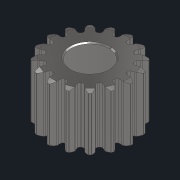
# Autodesk Inventor part: GEAHBB1_0-16-12-A-8_b
Saved by Autodesk Inventor 2022 (Build 260153000, 153)
## iProperties
Category: PARTsolutions
Company: MISUMI
Part Number: GEAHBB1_0-16-12-A-8_b
Material: 鋼、炭素鋼
Catalog Web Link: www.cadenas.de
Description: GEAHB1.0, GEAHBB1.0, GEAHBG1.0, GEAHS1.0, GEAB1.0, GEABB1.0, GEABG1.0, GEAS1.0, GEAKB1.0, GEAKBB1.0, GEAKBG1.0, GEAKS1.0_body-Spur Gears - Pressure Angle 20 Degree Module 1.0
Vendor: MISUMI
Document SubType Name: Modeling
Designer: partserver
Manufacturer: MISUMI
Mass: 13.5515 g
Surface Area: 17.3975 cm^2
Volume: 1.72631 cm^3
Density: 7.85 g/cm^3
Appearance: 半つや出し
PSOL_IDENT_0: {$CADENAS_DATA\23d-libs\misumi\metric\54_spur_gears\geab10\geab10.prj},528 {VTYP=3D},{NB=GEAHBB1.0-1
PSOL_IDENT_1: 6-12-A-8_b},{LINA=GEAHBB1.0-16-12-A-8},{NN=GEAHB1.0, GEAHBB1.0, GEAHBG1.0, GEAHS1.0, GEAB1.0, GEABB1
PSOL_IDENT_2: .0, GEABG1.0, GEAS1.0, GEAKB1.0, GEAKBB1.0, GEAKBG1.0, GEAKS1.0_body},{DATE=07.06.2021 01:25:53},{GE
PSOL_IDENT_3: OMDATE=08.04.2021 05:23:06},{VERSION=},{LINEID=20},{WBVAR=SHS,MAT,ST,NT,B,TSSE,TS,PS,ALT1,ALT2,TPC,A
PSOL_IDENT_4: LT11,ALT10,BS,ALT4,Z,J,ALT5,Q,R,S,T,ALT9,SRG,ALT6,LFC,LTC,MALT6,ALT7,KFC,KTC,K,ALT3,DIRALT3,QFC,QTC,
PSOL_IDENT_5: MALT3,ALT8,DIRALT8,ZFC,ZTC,U},{WBNUMERIC=NT,B,BS,Z,J,Q,R,S,T,SRG,LFC,LTC,KFC,KTC,K,QFC,QTC,ZFC,ZTC,U
PSOL_IDENT_6: }  {NB=GEAHBB1.0-16-12-A-8_b},{LINA=GEAHBB1.0-16-12-A-8},{KT=DUMMY},{PN=GEAHBB1.0-16-12-A-8},{SHS=RH
PSOL_IDENT_7: },{TYPE=GEAHBB},{MAT=S45C},{MATALG= 'S45C','S45C Equivalent','SUS304','SUS304' },{ST=BO},{STALG= '','
PSOL_IDENT_8: -','BO','Black Oxide','ENP','Electroless Nickel Plating'},{AC=-},{MOD=1.0},{NT=16},{NTALG=12,13,14,1
PSOL_IDENT_9: 5,16,17,18,19,20,21,22,23,24,25,26,27,28,29,30,32,33,34,35,36,38,39,40,42,44,45,46,48,49,50,51,52,54
PSOL_IDENT_10: ,55,56,57,58,60,62,63,64,65,66,68,69,70,72,75,76,77,78,80,81,84,85,88,90,91,92,95,96,98,99,100,110,1
PSOL_IDENT_11: 20},{B=12},{BALG=6,8,10,12},{TSSE=TSSE},{TSSEALG= '','Not Specified','TSSE','Specified'},{TS=A},{TSA
PSOL_IDENT_12: LG='K','K','A','A'},{TSPN=-A},{PS=8},{PSALG='6','6','6.35','6.35','7','7','8','8','9','9','10','10','
PSOL_IDENT_13: 11','11','12','12'},{P=8.00},{DD=16},{D=18},{G=13.5},{H=0},{L=0},{LL1=0},{LL2=0},{M=-},{ML=0.000},{A
PSOL_IDENT_14: LT1=},{ALT1ALG= '','N/A' },{ALT1PN=},{KC=0},{ALT2=},{ALT2ALG= '','N/A' },{TPC=N/A},{TPCALG= 'N/A' },
PSOL_IDENT_15: {ALT2PN=},{ALT11=},{ALT11ALG= '','N/A' },{ALT11PN=},{DEG=0},{ALT10=},{ALT10ALG= '','Not applicable'
PSOL_IDENT_16: },{BS=0.0},{BSALG=0},{BSMIN=3},{BSMAX=0},{ALT10PN=},{LL13D=0},{LL23D=0},{LBS=12},{ALT4=},{ALT4ALG=''
PSOL_IDENT_17: ,'Not applicable'},{ALT41=0},{ALT42=0},{ALT4PN=},{Z=0},{ZALG=0},{ZPN=},{ZMINL=10},{ZMAXL=9},{ZMINR=1
PSOL_IDENT_18: 0},{ZMAXR=9},{J=0.0},{JALG=0},{JPN=},{JMIN=2.0},{JMAX=0.0},{ALT5=},{ALT5ALG= '','Not applicable' },{
PSOL_IDENT_19: ALT5PN=},{Q=0},{QALG=0},{QPN=},{QMIN=10},{QMAX=9},{R=0},{RALG=0},{RPN=},{RMIN=10},{RMAX=9.0},{S=0},{
PSOL_IDENT_20: SALG=0},{SPN=},{SMIN=3},{SMAX=6},{T=0},{TALG=0},{TPN=},{TMIN=3},{TMAX=0},{ALT9=},{ALT9ALG= '','Not a
PSOL_IDENT_21: pplicable' },{SRG=0.0},{SRGALG=0},{SRGMIN=3.500},{SRGMINALG=3.500},{SRGMAX=0.000},{SRGMAXALG=0.000},
PSOL_IDENT_22: {DD2=0.0},{MM=0.00},{NN=0.00},{DD2ALG=0.000},{MMALG=0.000},{NNALG=0.000},{ALT9PN=},{ALT6=},{ALT6ALG=
PSOL_IDENT_23: '','Not applicable' },{ALT6PN=},{LFC=0},{LFCALG=0},{LTC=0},{LTCALG=0},{LPCDMIN=16},{LPCDMAX=6},{MAL
PSOL_IDENT_24: T6=N/A},{MALT6ALG= 'N/A' },{C=0.0},{ALT7=},{ALT7ALG= '','Not applicable' },{ALT7PN=},{KFC=0},{KFCALG=
PSOL_IDENT_25: [0]},{KTC=0},{KTCALG=[0]},{KPCDMIN1=15},{KPCDMAX1=-7},{KPCDMIN2=7},{KPCDMAX2=6},{KPCD=0},{K=0.0},{KA
PSOL_IDENT_26: LG=[0]},{KALT7L=12},{SCREW=0},{SCREWL=0},{ALT3=},{ALT3ALG= '','Not applicable' },{DIRALT3=},{DIRALT3
PSOL_IDENT_27: ALG= '','N/A' },{ALT3PN=},{QFC=0},{QFCALG=[0]},{QTC=0},{QTCALG=[0]},{QPCDMIN1=15},{QPCDMAX1=-7},{QPC
PSOL_IDENT_28: DMIN2=7},{QPCDMAX2=6},{CIFMALT3=3},{QPCD=0},{MALT3=N/A},{MALT3ALG= 'N/A' },{MALT3L=0},{MS1=3},{PITCH=
PSOL_IDENT_29: 0},{BB=3},{TT=0},{ALT8=},{ALT8ALG= '','Not applicable' },{DIRALT8=},{DIRALT8ALG= '','N/A' },{ALT8PN=
PSOL_IDENT_30: },{ZFC=0},{ZFCALG=[0]},{ZFCMIN=18},{ZFCMAX=3},{ZTC=0},{ZTCALG=[0]},{ZPCDMIN1=18},{ZPCDMIN2=11},{ZPCD
PSOL_IDENT_31: MAX1=-10},{ZPCDMAX2=3},{ZPCD=0},{U=0},{UALG=[0]},{UMAX=0},{UMAX1=0},{UMAX2=5},{UMIN=3},{U1=0.0},{U2=
PSOL_IDENT_32: 0.0},{F=0.0},{PLANE=4},{BL1=12},{BL2=11.5},{PCD=0},{SHN=0},{SHDEG1=0},{SHDEG2=0},{PZQRDD2=8},{ALT3LB
PSOL_IDENT_33: S=11.5},{D1=5.625},{D2=11.25},{D3=20},{D4=0.1},{D5=2.666667},{D6=2.461538},{D7=0.85},{D8=0.5},{D9=0.
PSOL_IDENT_34: 809481},{S1=15},{S2=1},{KR=22.5}
NB: GEAHBB1.0-16-12-A-8_b
NN: 0
NT: 16
NBSYN: $PN._b
LINA: GEAHBB1.0-16-12-A-8
CATALOG: Misumi
PN: GEAHBB1.0-16-12-A-8
SHS: Round Hole
MAT: S45C Equivalent
ST: Black Oxide
AC: -
MOD: 1
B: 12
TSSE: Specified
TS: A
PS: 8
DD: 16
D: 18
G: 13.5
H: 0
L: 0
LL1: 0
LL2: 0
M: -
ALT1: N/A
ALT2: N/A
TPC: N/A
ALT11: N/A
ALT10: Not applicable
BS: 0
ALT4: Not applicable
Z: 0
J: 0
ALT5: Not applicable
Q: 0
R: 0
S: 0
T: 0
ALT9: Not applicable
SRG: 0
DD2: 0
MM: 0
ALT6: Not applicable
LFC: 0
LTC: 0
MALT6: N/A
C: 0
ALT7: Not applicable
KFC: 0
KTC: 0
K: 0
ALT3: Not applicable
DIRALT3: N/A
QFC: 0
QTC: 0
MALT3: N/A
ALT8: Not applicable
DIRALT8: N/A
ZFC: 0
ZTC: 0
U: 0
U1: 0
U2: 0
F: 0
SUPPLIER: MISUMI
ARTICLENO: GEAHBB1.0-16-12-A-8_b
BOMINFO: GEAHBB1.0-16-12-A-8
CREATOR: CADENAS GmbH
Title: GEAHBB1.0-16-12-A-8
Author: Cadenas PARTsolutions
Comments: Spur Gears - Pressure Angle 20 Degree Module 1.0
Autodesk Inventor part; units mm, degrees
sketch "Sketch_12" plane through (0, 0, 0) normal (1, 0, 0) x (0, 1, 0)
  line L0 (0, 0) -> (0, 12)
  line L1 (0, 12) -> (8, 12)
  line L2 (8, 12) -> (14, 10.3923)
  line L3 (14, 10.3923) -> (14, 1.6077)
  line L4 (14, 1.6077) -> (8, 0)
  line L5 (8, 0) -> (0, 0)
  line L6 (0, 0) -> (0, 12)
  constraints: 14 end point
revolve "Revolution1" add sketch "Sketch_12" angle 360 about axis through (0, 0, 0) along (0, 0, -1)
sketch "Sketch_3" plane through (0, 0, 0) normal (0, 0, 1) x (1, 0, 0)
  circle A0 centre (0, 0) radius 36
  arc A1 (-8.9975, 0.2118) -> (-8.9975, -0.2118) centre (0, 0) ccw
  arc A2 (-8.9975, -0.2118) -> (-8.9598, -0.2877) centre (-8.8975, -0.2094) ccw
  arc A3 (-8.9598, -0.2877) -> (-7.9615, -0.7841) centre (-7.2994, 1.799) ccw
  arc A4 (-7.9615, -0.7841) -> (-7.6733, -0.8048) centre (-7.7605, 0) ccw
  arc A5 (-7.06, -0.8151) -> (-7.6733, -0.8048) centre (-7.4079, -3.252) ccw
  arc A6 (-6.6389, -1.2198) -> (-7.06, -0.8151) centre (-7.1306, -1.3101) ccw
  arc A7 (-6.6389, -1.2198) -> (-6.6003, -1.4137) centre (0, 0) ccw
  arc A8 (-6.8345, -1.9486) -> (-6.6003, -1.4137) centre (-7.0892, -1.5184) ccw
  arc A9 (-7.3971, -2.1929) -> (-6.8345, -1.9486) centre (-8.0885, 0.1695) ccw
  arc A10 (-7.3971, -2.1929) -> (-7.6555, -2.3223) centre (-7.1698, -2.9698) ccw
  arc A11 (-7.6555, -2.3223) -> (-8.3879, -3.163) centre (-6.0553, -4.4555) ccw
  arc A12 (-8.3879, -3.163) -> (-8.3936, -3.2476) centre (-8.3004, -3.2115) ccw
  arc A13 (-8.3936, -3.2476) -> (-8.2316, -3.6388) centre (0, 0) ccw
  arc A14 (-8.2316, -3.6388) -> (-8.1677, -3.6945) centre (-8.1401, -3.5984) ccw
  arc A15 (-8.1677, -3.6945) -> (-7.0554, -3.7712) centre (-7.4323, -1.1313) ccw
  arc A16 (-7.0554, -3.7712) -> (-6.7812, -3.6799) centre (-7.1698, -2.9698) ccw
  arc A17 (-6.2106, -3.4548) -> (-6.7812, -3.6799) centre (-5.5995, -5.8393) ccw
  arc A18 (-5.6667, -3.6675) -> (-6.2106, -3.4548) centre (-6.0865, -3.9392) ccw
  arc A19 (-5.6667, -3.6675) -> (-5.5569, -3.8319) centre (0, 0) ccw
  arc A20 (-5.5685, -4.4158) -> (-5.5569, -3.8319) centre (-5.9685, -4.1157) ccw
  arc A21 (-5.9949, -4.8568) -> (-5.5685, -4.4158) centre (-7.5377, -2.9387) ccw
  arc A22 (-5.9949, -4.8568) -> (-6.1841, -5.0751) centre (-5.4875, -5.4875) ccw
  arc A23 (-6.1841, -5.0751) -> (-6.5389, -6.1321) centre (-3.8894, -6.4336) ccw
  arc A24 (-6.5389, -6.1321) -> (-6.5119, -6.2125) centre (-6.4396, -6.1434) ccw
  arc A25 (-6.5119, -6.2125) -> (-6.2125, -6.5119) centre (0, 0) ccw
  arc A26 (-6.2125, -6.5119) -> (-6.1321, -6.5389) centre (-6.1434, -6.4396) ccw
  arc A27 (-6.1321, -6.5389) -> (-5.0751, -6.1841) centre (-6.4336, -3.8894) ccw
  arc A28 (-5.0751, -6.1841) -> (-4.8568, -5.9949) centre (-5.4875, -5.4875) ccw
  arc A29 (-4.4158, -5.5685) -> (-4.8568, -5.9949) centre (-2.9387, -7.5377) ccw
  arc A30 (-3.8319, -5.5569) -> (-4.4158, -5.5685) centre (-4.1157, -5.9685) ccw
  arc A31 (-3.8319, -5.5569) -> (-3.6675, -5.6667) centre (0, 0) ccw
  arc A32 (-3.4548, -6.2106) -> (-3.6675, -5.6667) centre (-3.9392, -6.0865) ccw
  arc A33 (-3.6799, -6.7812) -> (-3.4548, -6.2106) centre (-5.8393, -5.5995) ccw
  arc A34 (-3.6799, -6.7812) -> (-3.7712, -7.0554) centre (-2.9698, -7.1698) ccw
  arc A35 (-3.7712, -7.0554) -> (-3.6945, -8.1677) centre (-1.1313, -7.4323) ccw
  arc A36 (-3.6945, -8.1677) -> (-3.6388, -8.2316) centre (-3.5984, -8.1401) ccw
  arc A37 (-3.6388, -8.2316) -> (-3.2476, -8.3936) centre (0, 0) ccw
  arc A38 (-3.2476, -8.3936) -> (-3.163, -8.3879) centre (-3.2115, -8.3004) ccw
  arc A39 (-3.163, -8.3879) -> (-2.3223, -7.6555) centre (-4.4555, -6.0553) ccw
  arc A40 (-2.3223, -7.6555) -> (-2.1929, -7.3971) centre (-2.9698, -7.1698) ccw
  arc A41 (-1.9486, -6.8345) -> (-2.1929, -7.3971) centre (0.1695, -8.0885) ccw
  arc A42 (-1.4137, -6.6003) -> (-1.9486, -6.8345) centre (-1.5184, -7.0892) ccw
  arc A43 (-1.4137, -6.6003) -> (-1.2198, -6.6389) centre (0, 0) ccw
  arc A44 (-0.8151, -7.06) -> (-1.2198, -6.6389) centre (-1.3101, -7.1306) ccw
  arc A45 (-0.8048, -7.6733) -> (-0.8151, -7.06) centre (-3.252, -7.4079) ccw
  arc A46 (-0.8048, -7.6733) -> (-0.7841, -7.9615) centre (0, -7.7605) ccw
  arc A47 (-0.7841, -7.9615) -> (-0.2877, -8.9598) centre (1.799, -7.2994) ccw
  arc A48 (-0.2877, -8.9598) -> (-0.2118, -8.9975) centre (-0.2094, -8.8975) ccw
  arc A49 (-0.2118, -8.9975) -> (0.2118, -8.9975) centre (0, 0) ccw
  arc A50 (0.2118, -8.9975) -> (0.2877, -8.9598) centre (0.2094, -8.8975) ccw
  arc A51 (0.2877, -8.9598) -> (0.7841, -7.9615) centre (-1.799, -7.2994) ccw
  arc A52 (0.7841, -7.9615) -> (0.8048, -7.6733) centre (0, -7.7605) ccw
  arc A53 (0.8151, -7.06) -> (0.8048, -7.6733) centre (3.252, -7.4079) ccw
  arc A54 (1.2198, -6.6389) -> (0.8151, -7.06) centre (1.3101, -7.1306) ccw
  arc A55 (1.2198, -6.6389) -> (1.4137, -6.6003) centre (0, 0) ccw
  arc A56 (1.9486, -6.8345) -> (1.4137, -6.6003) centre (1.5184, -7.0892) ccw
  arc A57 (2.1929, -7.3971) -> (1.9486, -6.8345) centre (-0.1695, -8.0885) ccw
  arc A58 (2.1929, -7.3971) -> (2.3223, -7.6555) centre (2.9698, -7.1698) ccw
  arc A59 (2.3223, -7.6555) -> (3.163, -8.3879) centre (4.4555, -6.0553) ccw
  arc A60 (3.163, -8.3879) -> (3.2476, -8.3936) centre (3.2115, -8.3004) ccw
  arc A61 (3.2476, -8.3936) -> (3.6388, -8.2316) centre (0, 0) ccw
  arc A62 (3.6388, -8.2316) -> (3.6945, -8.1677) centre (3.5984, -8.1401) ccw
  arc A63 (3.6945, -8.1677) -> (3.7712, -7.0554) centre (1.1313, -7.4323) ccw
  arc A64 (3.7712, -7.0554) -> (3.6799, -6.7812) centre (2.9698, -7.1698) ccw
  arc A65 (3.4548, -6.2106) -> (3.6799, -6.7812) centre (5.8393, -5.5995) ccw
  arc A66 (3.6675, -5.6667) -> (3.4548, -6.2106) centre (3.9392, -6.0865) ccw
  arc A67 (3.6675, -5.6667) -> (3.8319, -5.5569) centre (0, 0) ccw
  arc A68 (4.4158, -5.5685) -> (3.8319, -5.5569) centre (4.1157, -5.9685) ccw
  arc A69 (4.8568, -5.9949) -> (4.4158, -5.5685) centre (2.9387, -7.5377) ccw
  arc A70 (4.8568, -5.9949) -> (5.0751, -6.1841) centre (5.4875, -5.4875) ccw
  arc A71 (5.0751, -6.1841) -> (6.1321, -6.5389) centre (6.4336, -3.8894) ccw
  arc A72 (6.1321, -6.5389) -> (6.2125, -6.5119) centre (6.1434, -6.4396) ccw
  arc A73 (6.2125, -6.5119) -> (6.5119, -6.2125) centre (0, 0) ccw
  arc A74 (6.5119, -6.2125) -> (6.5389, -6.1321) centre (6.4396, -6.1434) ccw
  arc A75 (6.5389, -6.1321) -> (6.1841, -5.0751) centre (3.8894, -6.4336) ccw
  arc A76 (6.1841, -5.0751) -> (5.9949, -4.8568) centre (5.4875, -5.4875) ccw
  arc A77 (5.5685, -4.4158) -> (5.9949, -4.8568) centre (7.5377, -2.9387) ccw
  arc A78 (5.5569, -3.8319) -> (5.5685, -4.4158) centre (5.9685, -4.1157) ccw
  arc A79 (5.5569, -3.8319) -> (5.6667, -3.6675) centre (0, 0) ccw
  arc A80 (6.2106, -3.4548) -> (5.6667, -3.6675) centre (6.0865, -3.9392) ccw
  arc A81 (6.7812, -3.6799) -> (6.2106, -3.4548) centre (5.5995, -5.8393) ccw
  arc A82 (6.7812, -3.6799) -> (7.0554, -3.7712) centre (7.1698, -2.9698) ccw
  arc A83 (7.0554, -3.7712) -> (8.1677, -3.6945) centre (7.4323, -1.1313) ccw
  arc A84 (8.1677, -3.6945) -> (8.2316, -3.6388) centre (8.1401, -3.5984) ccw
  arc A85 (8.2316, -3.6388) -> (8.3936, -3.2476) centre (0, 0) ccw
  arc A86 (8.3936, -3.2476) -> (8.3879, -3.163) centre (8.3004, -3.2115) ccw
  arc A87 (8.3879, -3.163) -> (7.6555, -2.3223) centre (6.0553, -4.4555) ccw
  arc A88 (7.6555, -2.3223) -> (7.3971, -2.1929) centre (7.1698, -2.9698) ccw
  arc A89 (6.8345, -1.9486) -> (7.3971, -2.1929) centre (8.0885, 0.1695) ccw
  arc A90 (6.6003, -1.4137) -> (6.8345, -1.9486) centre (7.0892, -1.5184) ccw
  arc A91 (6.6003, -1.4137) -> (6.6389, -1.2198) centre (0, 0) ccw
  arc A92 (7.06, -0.8151) -> (6.6389, -1.2198) centre (7.1306, -1.3101) ccw
  arc A93 (7.6733, -0.8048) -> (7.06, -0.8151) centre (7.4079, -3.252) ccw
  arc A94 (7.6733, -0.8048) -> (7.9615, -0.7841) centre (7.7605, 0) ccw
  arc A95 (7.9615, -0.7841) -> (8.9598, -0.2877) centre (7.2994, 1.799) ccw
  arc A96 (8.9598, -0.2877) -> (8.9975, -0.2118) centre (8.8975, -0.2094) ccw
  arc A97 (8.9975, -0.2118) -> (8.9975, 0.2118) centre (0, 0) ccw
  arc A98 (8.9975, 0.2118) -> (8.9598, 0.2877) centre (8.8975, 0.2094) ccw
  arc A99 (8.9598, 0.2877) -> (7.9615, 0.7841) centre (7.2994, -1.799) ccw
  arc A100 (7.9615, 0.7841) -> (7.6733, 0.8048) centre (7.7605, 0) ccw
  arc A101 (7.06, 0.8151) -> (7.6733, 0.8048) centre (7.4079, 3.252) ccw
  arc A102 (6.6389, 1.2198) -> (7.06, 0.8151) centre (7.1306, 1.3101) ccw
  arc A103 (6.6389, 1.2198) -> (6.6003, 1.4137) centre (0, 0) ccw
  arc A104 (6.8345, 1.9486) -> (6.6003, 1.4137) centre (7.0892, 1.5184) ccw
  arc A105 (7.3971, 2.1929) -> (6.8345, 1.9486) centre (8.0885, -0.1695) ccw
  arc A106 (7.3971, 2.1929) -> (7.6555, 2.3223) centre (7.1698, 2.9698) ccw
  arc A107 (7.6555, 2.3223) -> (8.3879, 3.163) centre (6.0553, 4.4555) ccw
  arc A108 (8.3879, 3.163) -> (8.3936, 3.2476) centre (8.3004, 3.2115) ccw
  arc A109 (8.3936, 3.2476) -> (8.2316, 3.6388) centre (0, 0) ccw
  arc A110 (8.2316, 3.6388) -> (8.1677, 3.6945) centre (8.1401, 3.5984) ccw
  arc A111 (8.1677, 3.6945) -> (7.0554, 3.7712) centre (7.4323, 1.1313) ccw
  arc A112 (7.0554, 3.7712) -> (6.7812, 3.6799) centre (7.1698, 2.9698) ccw
  arc A113 (6.2106, 3.4548) -> (6.7812, 3.6799) centre (5.5995, 5.8393) ccw
  arc A114 (5.6667, 3.6675) -> (6.2106, 3.4548) centre (6.0865, 3.9392) ccw
  arc A115 (5.6667, 3.6675) -> (5.5569, 3.8319) centre (0, 0) ccw
  arc A116 (5.5685, 4.4158) -> (5.5569, 3.8319) centre (5.9685, 4.1157) ccw
  arc A117 (5.9949, 4.8568) -> (5.5685, 4.4158) centre (7.5377, 2.9387) ccw
  arc A118 (5.9949, 4.8568) -> (6.1841, 5.0751) centre (5.4875, 5.4875) ccw
  arc A119 (6.1841, 5.0751) -> (6.5389, 6.1321) centre (3.8894, 6.4336) ccw
  arc A120 (6.5389, 6.1321) -> (6.5119, 6.2125) centre (6.4396, 6.1434) ccw
  arc A121 (6.5119, 6.2125) -> (6.2125, 6.5119) centre (0, 0) ccw
  arc A122 (6.2125, 6.5119) -> (6.1321, 6.5389) centre (6.1434, 6.4396) ccw
  arc A123 (6.1321, 6.5389) -> (5.0751, 6.1841) centre (6.4336, 3.8894) ccw
  arc A124 (5.0751, 6.1841) -> (4.8568, 5.9949) centre (5.4875, 5.4875) ccw
  arc A125 (4.4158, 5.5685) -> (4.8568, 5.9949) centre (2.9387, 7.5377) ccw
  arc A126 (3.8319, 5.5569) -> (4.4158, 5.5685) centre (4.1157, 5.9685) ccw
  arc A127 (3.8319, 5.5569) -> (3.6675, 5.6667) centre (0, 0) ccw
  arc A128 (3.4548, 6.2106) -> (3.6675, 5.6667) centre (3.9392, 6.0865) ccw
  arc A129 (3.6799, 6.7812) -> (3.4548, 6.2106) centre (5.8393, 5.5995) ccw
  arc A130 (3.6799, 6.7812) -> (3.7712, 7.0554) centre (2.9698, 7.1698) ccw
  arc A131 (3.7712, 7.0554) -> (3.6945, 8.1677) centre (1.1313, 7.4323) ccw
  arc A132 (3.6945, 8.1677) -> (3.6388, 8.2316) centre (3.5984, 8.1401) ccw
  arc A133 (3.6388, 8.2316) -> (3.2476, 8.3936) centre (0, 0) ccw
  arc A134 (3.2476, 8.3936) -> (3.163, 8.3879) centre (3.2115, 8.3004) ccw
  arc A135 (3.163, 8.3879) -> (2.3223, 7.6555) centre (4.4555, 6.0553) ccw
  arc A136 (2.3223, 7.6555) -> (2.1929, 7.3971) centre (2.9698, 7.1698) ccw
  arc A137 (1.9486, 6.8345) -> (2.1929, 7.3971) centre (-0.1695, 8.0885) ccw
  arc A138 (1.4137, 6.6003) -> (1.9486, 6.8345) centre (1.5184, 7.0892) ccw
  arc A139 (1.4137, 6.6003) -> (1.2198, 6.6389) centre (0, 0) ccw
  arc A140 (0.8151, 7.06) -> (1.2198, 6.6389) centre (1.3101, 7.1306) ccw
  arc A141 (0.8048, 7.6733) -> (0.8151, 7.06) centre (3.252, 7.4079) ccw
  arc A142 (0.8048, 7.6733) -> (0.7841, 7.9615) centre (0, 7.7605) ccw
  arc A143 (0.7841, 7.9615) -> (0.2877, 8.9598) centre (-1.799, 7.2994) ccw
  arc A144 (0.2877, 8.9598) -> (0.2118, 8.9975) centre (0.2094, 8.8975) ccw
  arc A145 (0.2118, 8.9975) -> (-0.2118, 8.9975) centre (0, 0) ccw
  arc A146 (-0.2118, 8.9975) -> (-0.2877, 8.9598) centre (-0.2094, 8.8975) ccw
  arc A147 (-0.2877, 8.9598) -> (-0.7841, 7.9615) centre (1.799, 7.2994) ccw
  arc A148 (-0.7841, 7.9615) -> (-0.8048, 7.6733) centre (0, 7.7605) ccw
  arc A149 (-0.8151, 7.06) -> (-0.8048, 7.6733) centre (-3.252, 7.4079) ccw
  arc A150 (-1.2198, 6.6389) -> (-0.8151, 7.06) centre (-1.3101, 7.1306) ccw
  arc A151 (-1.2198, 6.6389) -> (-1.4137, 6.6003) centre (0, 0) ccw
  arc A152 (-1.9486, 6.8345) -> (-1.4137, 6.6003) centre (-1.5184, 7.0892) ccw
  arc A153 (-2.1929, 7.3971) -> (-1.9486, 6.8345) centre (0.1695, 8.0885) ccw
  arc A154 (-2.1929, 7.3971) -> (-2.3223, 7.6555) centre (-2.9698, 7.1698) ccw
  arc A155 (-2.3223, 7.6555) -> (-3.163, 8.3879) centre (-4.4555, 6.0553) ccw
  arc A156 (-3.163, 8.3879) -> (-3.2476, 8.3936) centre (-3.2115, 8.3004) ccw
  arc A157 (-3.2476, 8.3936) -> (-3.6388, 8.2316) centre (0, 0) ccw
  arc A158 (-3.6388, 8.2316) -> (-3.6945, 8.1677) centre (-3.5984, 8.1401) ccw
  arc A159 (-3.6945, 8.1677) -> (-3.7712, 7.0554) centre (-1.1313, 7.4323) ccw
  arc A160 (-3.7712, 7.0554) -> (-3.6799, 6.7812) centre (-2.9698, 7.1698) ccw
  arc A161 (-3.4548, 6.2106) -> (-3.6799, 6.7812) centre (-5.8393, 5.5995) ccw
  arc A162 (-3.6675, 5.6667) -> (-3.4548, 6.2106) centre (-3.9392, 6.0865) ccw
  arc A163 (-3.6675, 5.6667) -> (-3.8319, 5.5569) centre (0, 0) ccw
  arc A164 (-4.4158, 5.5685) -> (-3.8319, 5.5569) centre (-4.1157, 5.9685) ccw
  arc A165 (-4.8568, 5.9949) -> (-4.4158, 5.5685) centre (-2.9387, 7.5377) ccw
  arc A166 (-4.8568, 5.9949) -> (-5.0751, 6.1841) centre (-5.4875, 5.4875) ccw
  arc A167 (-5.0751, 6.1841) -> (-6.1321, 6.5389) centre (-6.4336, 3.8894) ccw
  arc A168 (-6.1321, 6.5389) -> (-6.2125, 6.5119) centre (-6.1434, 6.4396) ccw
  arc A169 (-6.2125, 6.5119) -> (-6.5119, 6.2125) centre (0, 0) ccw
  arc A170 (-6.5119, 6.2125) -> (-6.5389, 6.1321) centre (-6.4396, 6.1434) ccw
  arc A171 (-6.5389, 6.1321) -> (-6.1841, 5.0751) centre (-3.8894, 6.4336) ccw
  arc A172 (-6.1841, 5.0751) -> (-5.9949, 4.8568) centre (-5.4875, 5.4875) ccw
  arc A173 (-5.5685, 4.4158) -> (-5.9949, 4.8568) centre (-7.5377, 2.9387) ccw
  arc A174 (-5.5569, 3.8319) -> (-5.5685, 4.4158) centre (-5.9685, 4.1157) ccw
  arc A175 (-5.5569, 3.8319) -> (-5.6667, 3.6675) centre (0, 0) ccw
  arc A176 (-6.2106, 3.4548) -> (-5.6667, 3.6675) centre (-6.0865, 3.9392) ccw
  arc A177 (-6.7812, 3.6799) -> (-6.2106, 3.4548) centre (-5.5995, 5.8393) ccw
  arc A178 (-6.7812, 3.6799) -> (-7.0554, 3.7712) centre (-7.1698, 2.9698) ccw
  arc A179 (-7.0554, 3.7712) -> (-8.1677, 3.6945) centre (-7.4323, 1.1313) ccw
  arc A180 (-8.1677, 3.6945) -> (-8.2316, 3.6388) centre (-8.1401, 3.5984) ccw
  arc A181 (-8.2316, 3.6388) -> (-8.3936, 3.2476) centre (0, 0) ccw
  arc A182 (-8.3936, 3.2476) -> (-8.3879, 3.163) centre (-8.3004, 3.2115) ccw
  arc A183 (-8.3879, 3.163) -> (-7.6555, 2.3223) centre (-6.0553, 4.4555) ccw
  arc A184 (-7.6555, 2.3223) -> (-7.3971, 2.1929) centre (-7.1698, 2.9698) ccw
  arc A185 (-6.8345, 1.9486) -> (-7.3971, 2.1929) centre (-8.0885, -0.1695) ccw
  arc A186 (-6.6003, 1.4137) -> (-6.8345, 1.9486) centre (-7.0892, 1.5184) ccw
  arc A187 (-6.6003, 1.4137) -> (-6.6389, 1.2198) centre (0, 0) ccw
  arc A188 (-7.06, 0.8151) -> (-6.6389, 1.2198) centre (-7.1306, 1.3101) ccw
  arc A189 (-7.6733, 0.8048) -> (-7.06, 0.8151) centre (-7.4079, 3.252) ccw
  arc A190 (-7.6733, 0.8048) -> (-7.9615, 0.7841) centre (-7.7605, 0) ccw
  arc A191 (-7.9615, 0.7841) -> (-8.9598, 0.2877) centre (-7.2994, -1.799) ccw
  arc A192 (-8.9598, 0.2877) -> (-8.9975, 0.2118) centre (-8.8975, 0.2094) ccw
  constraints: 384 point on circle, 193 centre point
extrude "Extrusion1" cut sketch "Sketch_3" along normal blind 13
sketch "Sketch3" plane through (0, 0, 0) normal (0, 0, -1) x (-1, 0, 0)
  point P0 (0, 0)
hole "Hole1" at (0, 0, 0) direction (0, 0, 1) diameter 8 depth 12
sketch "_____7" plane through (0, 0, 0) normal (1, 0, 0) x (0, 0, -1)
  line L0 (500, 0) -> (-500, 0)
  line L1 (-0.3, 4) -> (0, 4)
  line L2 (0, 4) -> (0, 4.3)
  line L3 (0, 4.3) -> (-0.3, 4)
  constraints: 8 end point
revolve "Revolution2" cut sketch "_____7" angle 360 about axis through (0, 0, -500) along (0, 0, -1)
sketch "_____17" plane through (0, 0, 0) normal (1, 0, 0) x (0, 0, -1)
  line L0 (500, 0) -> (-500, 0)
  line L1 (-12, 4.3) -> (-12, 4)
  line L2 (-12, 4) -> (-11.7, 4)
  line L3 (-11.7, 4) -> (-12, 4.3)
  constraints: 8 end point
revolve "Revolution3" cut sketch "_____17" angle 360 about axis through (0, 0, -500) along (0, 0, -1)
ref_plane "b_XY" through (0, 0, 0) normal (0, 0, 1) x (1, 0, 0)
ref_plane "b_YZ" through (0, 0, 0) normal (1, 0, 0) x (0, 1, 0)
ref_plane "b_ZX" through (0, 0, 0) normal (0, 1, 0) x (0, 0, 1)
ref_plane "turn_around_XY" through (0, 0, 0) normal (-1, 0, 0) x (0, 0, -1)
ref_plane "turn_around_YZ" through (0, 0, 0) normal (0, 0, -1) x (0, -1, 0)
ref_plane "turn_around_ZX" through (0, 0, 0) normal (0, -1, 0) x (-1, 0, 0)
sketch "スケッチ6" plane through (0, 0, 0) normal (0, 0, -1) x (-1, 0, 0)
  circle A0 centre (0, 0) radius 4.05
  dimension "d13" = 8.1
  constraints: 1 centre point, 1 coincident
  measures "d13" diameter of A0
extrude "押し出し2" cut sketch "スケッチ6" against normal through all
body "Solid1"
